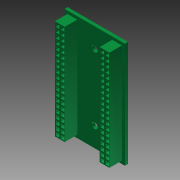
# Autodesk Inventor part: mbed breakout board
Saved by Autodesk Inventor 2012 (Build 160160000, 160)
## iProperties
Created: 2012-03-03
Part Number: mbed breakout board
Material: Default
Document SubType Name: Modeling
Designer: Lauszus
Density: 1 g/cm^3
Author: Lauszus
Autodesk Inventor part; units mm, degrees
ref_plane "YZ Plane" through (0, 0, 0) normal (1, 0, 0) x (0, 1, 0)
ref_plane "XZ Plane" through (0, 0, 0) normal (0, 1, 0) x (-1, 0, 0)
ref_plane "XY Plane" through (0, 0, 0) normal (0, 0, 1) x (1, 0, 0)
sketch "Sketch1" plane through (0, 0, 0) normal (0, 0, 1) x (1, 0, 0)
  line L0 (-19.1815, 31.3375) -> (11.6785, 31.3375)
  line L1 (11.6785, 31.3375) -> (11.6785, -22.6377)
  line L2 (11.6785, -22.6377) -> (-19.1815, -22.6377)
  line L3 (-19.1815, -22.6377) -> (-19.1815, 31.3375)
  line L4 (-17.6815, 29.8375) -> (-12.6815, 29.8375)
  line L5 (-12.6815, 29.8375) -> (-12.6815, -21.1377)
  line L6 (-12.6815, -21.1377) -> (-17.6815, -21.1377)
  line L7 (-17.6815, -21.1377) -> (-17.6815, 29.8375)
  line L8 (-17.1815, -20.6377) -> (-15.4815, -20.6377)
  line L9 (-15.4815, -20.6377) -> (-15.4815, -18.9377)
  line L10 (-15.4815, -18.9377) -> (-17.1815, -18.9377)
  line L11 (-17.1815, -18.9377) -> (-17.1815, -20.6377)
  line L12 (-14.6415, -20.6377) -> (-12.9415, -20.6377)
  line L13 (-12.9415, -20.6377) -> (-12.9415, -18.9377)
  line L14 (-12.9415, -18.9377) -> (-14.6415, -18.9377)
  line L15 (-14.6415, -18.9377) -> (-14.6415, -20.6377)
  line L16 (-17.1815, -18.0977) -> (-15.4815, -18.0977)
  line L17 (-15.4815, -18.0977) -> (-15.4815, -16.3977)
  line L18 (-15.4815, -16.3977) -> (-17.1815, -16.3977)
  line L19 (-17.1815, -16.3977) -> (-17.1815, -18.0977)
  line L20 (-14.6415, -18.0977) -> (-12.9415, -18.0977)
  line L21 (-12.9415, -18.0977) -> (-12.9415, -16.3977)
  line L22 (-12.9415, -16.3977) -> (-14.6415, -16.3977)
  line L23 (-14.6415, -16.3977) -> (-14.6415, -18.0977)
  line L24 (-17.1815, -15.5577) -> (-15.4815, -15.5577)
  line L25 (-15.4815, -15.5577) -> (-15.4815, -13.8577)
  line L26 (-15.4815, -13.8577) -> (-17.1815, -13.8577)
  line L27 (-17.1815, -13.8577) -> (-17.1815, -15.5577)
  line L28 (-14.6415, -15.5577) -> (-12.9415, -15.5577)
  line L29 (-12.9415, -15.5577) -> (-12.9415, -13.8577)
  line L30 (-12.9415, -13.8577) -> (-14.6415, -13.8577)
  line L31 (-14.6415, -13.8577) -> (-14.6415, -15.5577)
  line L32 (-12.9415, -11.3177) -> (-14.6415, -11.3177)
  line L33 (-12.9415, -13.0177) -> (-12.9415, -11.3177)
  line L34 (-14.6415, -11.3177) -> (-14.6415, -13.0177)
  line L35 (-14.6415, -13.0177) -> (-12.9415, -13.0177)
  line L36 (-17.1815, -13.0177) -> (-15.4815, -13.0177)
  line L37 (-15.4815, -13.0177) -> (-15.4815, -11.3177)
  line L38 (-15.4815, -11.3177) -> (-17.1815, -11.3177)
  line L39 (-17.1815, -11.3177) -> (-17.1815, -13.0177)
  line L40 (-17.1815, -10.4777) -> (-15.4815, -10.4777)
  line L41 (-15.4815, -10.4777) -> (-15.4815, -8.7777)
  line L42 (-15.4815, -8.7777) -> (-17.1815, -8.7777)
  line L43 (-17.1815, -8.7777) -> (-17.1815, -10.4777)
  line L44 (-14.6415, -10.4777) -> (-12.9415, -10.4777)
  line L45 (-12.9415, -10.4777) -> (-12.9415, -8.7777)
  line L46 (-12.9415, -8.7777) -> (-14.6415, -8.7777)
  line L47 (-14.6415, -8.7777) -> (-14.6415, -10.4777)
  line L48 (-12.9415, -6.2377) -> (-14.6415, -6.2377)
  line L49 (-12.9415, -7.9377) -> (-12.9415, -6.2377)
  line L50 (-14.6415, -6.2377) -> (-14.6415, -7.9377)
  line L51 (-14.6415, -7.9377) -> (-12.9415, -7.9377)
  line L52 (-17.1815, -7.9377) -> (-15.4815, -7.9377)
  line L53 (-15.4815, -7.9377) -> (-15.4815, -6.2377)
  line L54 (-15.4815, -6.2377) -> (-17.1815, -6.2377)
  line L55 (-17.1815, -6.2377) -> (-17.1815, -7.9377)
  line L56 (-17.1815, -5.3977) -> (-15.4815, -5.3977)
  line L57 (-15.4815, -5.3977) -> (-15.4815, -3.6977)
  line L58 (-15.4815, -3.6977) -> (-17.1815, -3.6977)
  line L59 (-17.1815, -3.6977) -> (-17.1815, -5.3977)
  line L60 (-14.6415, -5.3977) -> (-12.9415, -5.3977)
  line L61 (-12.9415, -5.3977) -> (-12.9415, -3.6977)
  line L62 (-12.9415, -3.6977) -> (-14.6415, -3.6977)
  line L63 (-14.6415, -3.6977) -> (-14.6415, -5.3977)
  line L64 (-12.9415, -1.1577) -> (-14.6415, -1.1577)
  line L65 (-12.9415, -2.8577) -> (-12.9415, -1.1577)
  line L66 (-14.6415, -1.1577) -> (-14.6415, -2.8577)
  line L67 (-14.6415, -2.8577) -> (-12.9415, -2.8577)
  line L68 (-17.1815, -2.8577) -> (-15.4815, -2.8577)
  line L69 (-15.4815, -2.8577) -> (-15.4815, -1.1577)
  line L70 (-15.4815, -1.1577) -> (-17.1815, -1.1577)
  line L71 (-17.1815, -1.1577) -> (-17.1815, -2.8577)
  line L72 (-17.1815, -0.3177) -> (-15.4815, -0.3177)
  line L73 (-15.4815, -0.3177) -> (-15.4815, 1.3823)
  line L74 (-15.4815, 1.3823) -> (-17.1815, 1.3823)
  line L75 (-17.1815, 1.3823) -> (-17.1815, -0.3177)
  line L76 (-14.6415, -0.3177) -> (-12.9415, -0.3177)
  line L77 (-12.9415, -0.3177) -> (-12.9415, 1.3823)
  line L78 (-12.9415, 1.3823) -> (-14.6415, 1.3823)
  line L79 (-14.6415, 1.3823) -> (-14.6415, -0.3177)
  line L80 (-12.9415, 3.9223) -> (-14.6415, 3.9223)
  line L81 (-12.9415, 2.2223) -> (-12.9415, 3.9223)
  line L82 (-14.6415, 3.9223) -> (-14.6415, 2.2223)
  line L83 (-14.6415, 2.2223) -> (-12.9415, 2.2223)
  line L84 (-17.1815, 2.2223) -> (-15.4815, 2.2223)
  line L85 (-15.4815, 2.2223) -> (-15.4815, 3.9223)
  line L86 (-15.4815, 3.9223) -> (-17.1815, 3.9223)
  line L87 (-17.1815, 3.9223) -> (-17.1815, 2.2223)
  line L88 (-17.1815, 4.7623) -> (-15.4815, 4.7623)
  line L89 (-15.4815, 4.7623) -> (-15.4815, 6.4623)
  line L90 (-15.4815, 6.4623) -> (-17.1815, 6.4623)
  line L91 (-17.1815, 6.4623) -> (-17.1815, 4.7623)
  line L92 (-14.6415, 4.7623) -> (-12.9415, 4.7623)
  line L93 (-12.9415, 4.7623) -> (-12.9415, 6.4623)
  line L94 (-12.9415, 6.4623) -> (-14.6415, 6.4623)
  line L95 (-14.6415, 6.4623) -> (-14.6415, 4.7623)
  line L96 (-12.9415, 9.0023) -> (-14.6415, 9.0023)
  line L97 (-12.9415, 7.3023) -> (-12.9415, 9.0023)
  line L98 (-14.6415, 9.0023) -> (-14.6415, 7.3023)
  line L99 (-14.6415, 7.3023) -> (-12.9415, 7.3023)
  line L100 (-17.1815, 7.3023) -> (-15.4815, 7.3023)
  line L101 (-15.4815, 7.3023) -> (-15.4815, 9.0023)
  line L102 (-15.4815, 9.0023) -> (-17.1815, 9.0023)
  line L103 (-17.1815, 9.0023) -> (-17.1815, 7.3023)
  line L104 (-17.1815, 9.8423) -> (-15.4815, 9.8423)
  line L105 (-15.4815, 9.8423) -> (-15.4815, 11.5423)
  line L106 (-15.4815, 11.5423) -> (-17.1815, 11.5423)
  line L107 (-17.1815, 11.5423) -> (-17.1815, 9.8423)
  line L108 (-14.6415, 9.8423) -> (-12.9415, 9.8423)
  line L109 (-12.9415, 9.8423) -> (-12.9415, 11.5423)
  line L110 (-12.9415, 11.5423) -> (-14.6415, 11.5423)
  line L111 (-14.6415, 11.5423) -> (-14.6415, 9.8423)
  line L112 (-12.9415, 14.0823) -> (-14.6415, 14.0823)
  line L113 (-12.9415, 12.3823) -> (-12.9415, 14.0823)
  line L114 (-14.6415, 14.0823) -> (-14.6415, 12.3823)
  line L115 (-14.6415, 12.3823) -> (-12.9415, 12.3823)
  line L116 (-17.1815, 12.3823) -> (-15.4815, 12.3823)
  line L117 (-15.4815, 12.3823) -> (-15.4815, 14.0823)
  line L118 (-15.4815, 14.0823) -> (-17.1815, 14.0823)
  line L119 (-17.1815, 14.0823) -> (-17.1815, 12.3823)
  line L120 (-17.1815, 14.9223) -> (-15.4815, 14.9223)
  line L121 (-15.4815, 14.9223) -> (-15.4815, 16.6223)
  line L122 (-15.4815, 16.6223) -> (-17.1815, 16.6223)
  line L123 (-17.1815, 16.6223) -> (-17.1815, 14.9223)
  line L124 (-14.6415, 14.9223) -> (-12.9415, 14.9223)
  line L125 (-12.9415, 14.9223) -> (-12.9415, 16.6223)
  line L126 (-12.9415, 16.6223) -> (-14.6415, 16.6223)
  line L127 (-14.6415, 16.6223) -> (-14.6415, 14.9223)
  line L128 (-12.9415, 19.1623) -> (-14.6415, 19.1623)
  line L129 (-12.9415, 17.4623) -> (-12.9415, 19.1623)
  line L130 (-14.6415, 19.1623) -> (-14.6415, 17.4623)
  line L131 (-14.6415, 17.4623) -> (-12.9415, 17.4623)
  line L132 (-17.1815, 17.4623) -> (-15.4815, 17.4623)
  line L133 (-15.4815, 17.4623) -> (-15.4815, 19.1623)
  line L134 (-15.4815, 19.1623) -> (-17.1815, 19.1623)
  line L135 (-17.1815, 19.1623) -> (-17.1815, 17.4623)
  line L136 (-17.1815, 20.0023) -> (-15.4815, 20.0023)
  line L137 (-15.4815, 20.0023) -> (-15.4815, 21.7023)
  line L138 (-15.4815, 21.7023) -> (-17.1815, 21.7023)
  line L139 (-17.1815, 21.7023) -> (-17.1815, 20.0023)
  line L140 (-14.6415, 20.0023) -> (-12.9415, 20.0023)
  line L141 (-12.9415, 20.0023) -> (-12.9415, 21.7023)
  line L142 (-12.9415, 21.7023) -> (-14.6415, 21.7023)
  line L143 (-14.6415, 21.7023) -> (-14.6415, 20.0023)
  line L144 (-12.9415, 24.2423) -> (-14.6415, 24.2423)
  line L145 (-12.9415, 22.5423) -> (-12.9415, 24.2423)
  line L146 (-14.6415, 24.2423) -> (-14.6415, 22.5423)
  line L147 (-14.6415, 22.5423) -> (-12.9415, 22.5423)
  line L148 (-17.1815, 22.5423) -> (-15.4815, 22.5423)
  line L149 (-15.4815, 22.5423) -> (-15.4815, 24.2423)
  line L150 (-15.4815, 24.2423) -> (-17.1815, 24.2423)
  line L151 (-17.1815, 24.2423) -> (-17.1815, 22.5423)
  line L152 (-17.1815, 25.0823) -> (-15.4815, 25.0823)
  line L153 (-15.4815, 25.0823) -> (-15.4815, 26.7823)
  line L154 (-15.4815, 26.7823) -> (-17.1815, 26.7823)
  line L155 (-17.1815, 26.7823) -> (-17.1815, 25.0823)
  line L156 (-14.6415, 25.0823) -> (-12.9415, 25.0823)
  line L157 (-12.9415, 25.0823) -> (-12.9415, 26.7823)
  line L158 (-12.9415, 26.7823) -> (-14.6415, 26.7823)
  line L159 (-14.6415, 26.7823) -> (-14.6415, 25.0823)
  line L160 (-12.9415, 29.3223) -> (-14.6415, 29.3223)
  line L161 (-12.9415, 27.6223) -> (-12.9415, 29.3223)
  line L162 (-14.6415, 29.3223) -> (-14.6415, 27.6223)
  line L163 (-14.6415, 27.6223) -> (-12.9415, 27.6223)
  line L164 (-17.1815, 27.6223) -> (-15.4815, 27.6223)
  line L165 (-15.4815, 27.6223) -> (-15.4815, 29.3223)
  line L166 (-15.4815, 29.3223) -> (-17.1815, 29.3223)
  line L167 (-17.1815, 29.3223) -> (-17.1815, 27.6223)
  line L168 (5.1785, 29.8375) -> (10.1785, 29.8375)
  line L169 (10.1785, 29.8375) -> (10.1785, -21.1377)
  line L170 (10.1785, -21.1377) -> (5.1785, -21.1377)
  line L171 (5.1785, -21.1377) -> (5.1785, 29.8375)
  line L172 (5.6785, -20.6377) -> (7.3785, -20.6377)
  line L173 (7.3785, -20.6377) -> (7.3785, -18.9377)
  line L174 (7.3785, -18.9377) -> (5.6785, -18.9377)
  line L175 (5.6785, -18.9377) -> (5.6785, -20.6377)
  line L176 (8.2185, -20.6377) -> (9.9185, -20.6377)
  line L177 (9.9185, -20.6377) -> (9.9185, -18.9377)
  line L178 (9.9185, -18.9377) -> (8.2185, -18.9377)
  line L179 (8.2185, -18.9377) -> (8.2185, -20.6377)
  line L180 (9.9185, -16.3977) -> (8.2185, -16.3977)
  line L181 (9.9185, -18.0977) -> (9.9185, -16.3977)
  line L182 (8.2185, -16.3977) -> (8.2185, -18.0977)
  line L183 (8.2185, -18.0977) -> (9.9185, -18.0977)
  line L184 (5.6785, -18.0977) -> (7.3785, -18.0977)
  line L185 (7.3785, -18.0977) -> (7.3785, -16.3977)
  line L186 (7.3785, -16.3977) -> (5.6785, -16.3977)
  line L187 (5.6785, -16.3977) -> (5.6785, -18.0977)
  line L188 (5.6785, -15.5577) -> (7.3785, -15.5577)
  line L189 (5.6785, -13.8577) -> (5.6785, -15.5577)
  line L190 (7.3785, -13.8577) -> (5.6785, -13.8577)
  line L191 (7.3785, -15.5577) -> (7.3785, -13.8577)
  line L192 (5.6785, -13.0177) -> (7.3785, -13.0177)
  line L193 (5.6785, -11.3177) -> (5.6785, -13.0177)
  line L194 (7.3785, -11.3177) -> (5.6785, -11.3177)
  line L195 (7.3785, -13.0177) -> (7.3785, -11.3177)
  line L196 (9.9185, -11.3177) -> (8.2185, -11.3177)
  line L197 (8.2185, -11.3177) -> (8.2185, -13.0177)
  line L198 (9.9185, -13.0177) -> (9.9185, -11.3177)
  line L199 (8.2185, -13.0177) -> (9.9185, -13.0177)
  line L200 (9.9185, -13.8577) -> (8.2185, -13.8577)
  line L201 (8.2185, -13.8577) -> (8.2185, -15.5577)
  line L202 (8.2185, -15.5577) -> (9.9185, -15.5577)
  line L203 (9.9185, -15.5577) -> (9.9185, -13.8577)
  line L204 (5.6785, -10.4777) -> (7.3785, -10.4777)
  line L205 (5.6785, -8.7777) -> (5.6785, -10.4777)
  line L206 (7.3785, -8.7777) -> (5.6785, -8.7777)
  line L207 (7.3785, -10.4777) -> (7.3785, -8.7777)
  line L208 (5.6785, -7.9377) -> (7.3785, -7.9377)
  line L209 (5.6785, -6.2377) -> (5.6785, -7.9377)
  line L210 (7.3785, -6.2377) -> (5.6785, -6.2377)
  line L211 (7.3785, -7.9377) -> (7.3785, -6.2377)
  line L212 (9.9185, -6.2377) -> (8.2185, -6.2377)
  line L213 (8.2185, -6.2377) -> (8.2185, -7.9377)
  line L214 (9.9185, -7.9377) -> (9.9185, -6.2377)
  line L215 (8.2185, -7.9377) -> (9.9185, -7.9377)
  line L216 (9.9185, -8.7777) -> (8.2185, -8.7777)
  line L217 (8.2185, -8.7777) -> (8.2185, -10.4777)
  line L218 (8.2185, -10.4777) -> (9.9185, -10.4777)
  line L219 (9.9185, -10.4777) -> (9.9185, -8.7777)
  line L220 (5.6785, -5.3977) -> (7.3785, -5.3977)
  line L221 (5.6785, -3.6977) -> (5.6785, -5.3977)
  line L222 (7.3785, -3.6977) -> (5.6785, -3.6977)
  line L223 (7.3785, -5.3977) -> (7.3785, -3.6977)
  line L224 (5.6785, -2.8577) -> (7.3785, -2.8577)
  line L225 (5.6785, -1.1577) -> (5.6785, -2.8577)
  line L226 (7.3785, -1.1577) -> (5.6785, -1.1577)
  line L227 (7.3785, -2.8577) -> (7.3785, -1.1577)
  line L228 (9.9185, -1.1577) -> (8.2185, -1.1577)
  line L229 (8.2185, -1.1577) -> (8.2185, -2.8577)
  line L230 (9.9185, -2.8577) -> (9.9185, -1.1577)
  line L231 (8.2185, -2.8577) -> (9.9185, -2.8577)
  line L232 (9.9185, -3.6977) -> (8.2185, -3.6977)
  line L233 (8.2185, -3.6977) -> (8.2185, -5.3977)
  line L234 (8.2185, -5.3977) -> (9.9185, -5.3977)
  line L235 (9.9185, -5.3977) -> (9.9185, -3.6977)
  line L236 (5.6785, -0.3177) -> (7.3785, -0.3177)
  line L237 (5.6785, 1.3823) -> (5.6785, -0.3177)
  line L238 (7.3785, 1.3823) -> (5.6785, 1.3823)
  line L239 (7.3785, -0.3177) -> (7.3785, 1.3823)
  line L240 (5.6785, 2.2223) -> (7.3785, 2.2223)
  line L241 (5.6785, 3.9223) -> (5.6785, 2.2223)
  line L242 (7.3785, 3.9223) -> (5.6785, 3.9223)
  line L243 (7.3785, 2.2223) -> (7.3785, 3.9223)
  line L244 (9.9185, 3.9223) -> (8.2185, 3.9223)
  line L245 (8.2185, 3.9223) -> (8.2185, 2.2223)
  line L246 (9.9185, 2.2223) -> (9.9185, 3.9223)
  line L247 (8.2185, 2.2223) -> (9.9185, 2.2223)
  line L248 (9.9185, 1.3823) -> (8.2185, 1.3823)
  line L249 (8.2185, 1.3823) -> (8.2185, -0.3177)
  line L250 (8.2185, -0.3177) -> (9.9185, -0.3177)
  line L251 (9.9185, -0.3177) -> (9.9185, 1.3823)
  line L252 (5.6785, 4.7623) -> (7.3785, 4.7623)
  line L253 (5.6785, 6.4623) -> (5.6785, 4.7623)
  line L254 (7.3785, 6.4623) -> (5.6785, 6.4623)
  line L255 (7.3785, 4.7623) -> (7.3785, 6.4623)
  line L256 (5.6785, 7.3023) -> (7.3785, 7.3023)
  line L257 (5.6785, 9.0023) -> (5.6785, 7.3023)
  line L258 (7.3785, 9.0023) -> (5.6785, 9.0023)
  line L259 (7.3785, 7.3023) -> (7.3785, 9.0023)
  line L260 (9.9185, 9.0023) -> (8.2185, 9.0023)
  line L261 (8.2185, 9.0023) -> (8.2185, 7.3023)
  line L262 (9.9185, 7.3023) -> (9.9185, 9.0023)
  line L263 (8.2185, 7.3023) -> (9.9185, 7.3023)
  line L264 (9.9185, 6.4623) -> (8.2185, 6.4623)
  line L265 (8.2185, 6.4623) -> (8.2185, 4.7623)
  line L266 (8.2185, 4.7623) -> (9.9185, 4.7623)
  line L267 (9.9185, 4.7623) -> (9.9185, 6.4623)
  line L268 (5.6785, 9.8423) -> (7.3785, 9.8423)
  line L269 (5.6785, 11.5423) -> (5.6785, 9.8423)
  line L270 (7.3785, 11.5423) -> (5.6785, 11.5423)
  line L271 (7.3785, 9.8423) -> (7.3785, 11.5423)
  line L272 (5.6785, 12.3823) -> (7.3785, 12.3823)
  line L273 (5.6785, 14.0823) -> (5.6785, 12.3823)
  line L274 (7.3785, 14.0823) -> (5.6785, 14.0823)
  line L275 (7.3785, 12.3823) -> (7.3785, 14.0823)
  line L276 (9.9185, 14.0823) -> (8.2185, 14.0823)
  line L277 (8.2185, 14.0823) -> (8.2185, 12.3823)
  line L278 (9.9185, 12.3823) -> (9.9185, 14.0823)
  line L279 (8.2185, 12.3823) -> (9.9185, 12.3823)
  line L280 (9.9185, 11.5423) -> (8.2185, 11.5423)
  line L281 (8.2185, 11.5423) -> (8.2185, 9.8423)
  line L282 (8.2185, 9.8423) -> (9.9185, 9.8423)
  line L283 (9.9185, 9.8423) -> (9.9185, 11.5423)
  line L284 (5.6785, 14.9223) -> (7.3785, 14.9223)
  line L285 (5.6785, 16.6223) -> (5.6785, 14.9223)
  line L286 (7.3785, 16.6223) -> (5.6785, 16.6223)
  line L287 (7.3785, 14.9223) -> (7.3785, 16.6223)
  line L288 (5.6785, 17.4623) -> (7.3785, 17.4623)
  line L289 (5.6785, 19.1623) -> (5.6785, 17.4623)
  line L290 (7.3785, 19.1623) -> (5.6785, 19.1623)
  line L291 (7.3785, 17.4623) -> (7.3785, 19.1623)
  line L292 (9.9185, 19.1623) -> (8.2185, 19.1623)
  line L293 (8.2185, 19.1623) -> (8.2185, 17.4623)
  line L294 (9.9185, 17.4623) -> (9.9185, 19.1623)
  line L295 (8.2185, 17.4623) -> (9.9185, 17.4623)
  line L296 (9.9185, 16.6223) -> (8.2185, 16.6223)
  line L297 (8.2185, 16.6223) -> (8.2185, 14.9223)
  line L298 (8.2185, 14.9223) -> (9.9185, 14.9223)
  line L299 (9.9185, 14.9223) -> (9.9185, 16.6223)
  line L300 (5.6785, 20.0023) -> (7.3785, 20.0023)
  line L301 (5.6785, 21.7023) -> (5.6785, 20.0023)
  line L302 (7.3785, 21.7023) -> (5.6785, 21.7023)
  line L303 (7.3785, 20.0023) -> (7.3785, 21.7023)
  line L304 (5.6785, 22.5423) -> (7.3785, 22.5423)
  line L305 (5.6785, 24.2423) -> (5.6785, 22.5423)
  line L306 (7.3785, 24.2423) -> (5.6785, 24.2423)
  line L307 (7.3785, 22.5423) -> (7.3785, 24.2423)
  line L308 (9.9185, 24.2423) -> (8.2185, 24.2423)
  line L309 (8.2185, 24.2423) -> (8.2185, 22.5423)
  line L310 (9.9185, 22.5423) -> (9.9185, 24.2423)
  line L311 (8.2185, 22.5423) -> (9.9185, 22.5423)
  line L312 (9.9185, 21.7023) -> (8.2185, 21.7023)
  line L313 (8.2185, 21.7023) -> (8.2185, 20.0023)
  line L314 (8.2185, 20.0023) -> (9.9185, 20.0023)
  line L315 (9.9185, 20.0023) -> (9.9185, 21.7023)
  line L316 (5.6785, 25.0823) -> (7.3785, 25.0823)
  line L317 (5.6785, 26.7823) -> (5.6785, 25.0823)
  line L318 (7.3785, 26.7823) -> (5.6785, 26.7823)
  line L319 (7.3785, 25.0823) -> (7.3785, 26.7823)
  line L320 (5.6785, 27.6223) -> (7.3785, 27.6223)
  line L321 (5.6785, 29.3223) -> (5.6785, 27.6223)
  line L322 (7.3785, 29.3223) -> (5.6785, 29.3223)
  line L323 (7.3785, 27.6223) -> (7.3785, 29.3223)
  line L324 (9.9185, 29.3223) -> (8.2185, 29.3223)
  line L325 (8.2185, 29.3223) -> (8.2185, 27.6223)
  line L326 (9.9185, 27.6223) -> (9.9185, 29.3223)
  line L327 (8.2185, 27.6223) -> (9.9185, 27.6223)
  line L328 (9.9185, 26.7823) -> (8.2185, 26.7823)
  line L329 (8.2185, 26.7823) -> (8.2185, 25.0823)
  line L330 (8.2185, 25.0823) -> (9.9185, 25.0823)
  line L331 (9.9185, 25.0823) -> (9.9185, 26.7823)
  circle A0 centre (-3.7515, 21.3375) radius 1.5
  circle A1 centre (-3.7515, -12.6377) radius 1.5
  point P0 (0, 0)
  dimension "d3" = 50.9753
  dimension "d4" = 5
  dimension "d5" = 1.5
  dimension "d6" = 1.5
  dimension "d7" = 1.7
  dimension "d8" = 1.7
  dimension "d9" = 2.54
  dimension "d10" = 1.7
  dimension "d11" = 1.7
  dimension "d12" = 0.5
  dimension "d13" = 0.5
  dimension "d14" = 0.5
  dimension "d15" = 1.7
  dimension "d16" = 1.7
  dimension "d17" = 2.54
  dimension "d18" = 1.7
  dimension "d19" = 1.7
  dimension "d21" = 2.54
  dimension "d22" = 2.54
  dimension "d23" = 0.5
  dimension "d26" = 5.08
  dimension "d33" = 22.86
  dimension "d38" = 1.5
  dimension "d39" = 1.5
  dimension "d40" = 15.43
  dimension "d41" = 15.43
  dimension "d42" = 10
  dimension "d43" = 10
  dimension "d44" = 3
  dimension "d45" = 3
  constraints: 664 end point, 12 parallel, 7 horizontal, 6 perpendicular, 2 centre point, 1 vertical, 616 other
  measures "d3" distance of L4.end L5.end
  measures "d4" distance of L4.start L4.end
  measures "d5" distance between parallel lines of L2 L6
  measures "d6" distance between parallel lines of L3 L7
  measures "d7" distance of L10.end L8.start
  measures "d8" distance of L9.end L10.end
  measures "d9" distance between parallel lines of L11 L15
  measures "d10" distance of L14.end L12.start
  measures "d11" distance of L13.end L14.end
  measures "d12" distance between parallel lines of L7 L11
  measures "d13" distance between parallel lines of L6 L8
  measures "d14" distance between parallel lines of L6 L12
  measures "d15" distance of L18.end L16.start
  measures "d16" distance of L17.end L18.end
  measures "d17" distance between parallel lines of L19 L23
  measures "d18" distance of L22.end L23.end
  measures "d19" distance of L22.start L22.end
  measures "d21" distance between parallel lines of L8 L16
  measures "d22" distance between parallel lines of L12 L20
  measures "d23" distance between parallel lines of L7 L19
  measures "d26" distance of L8.start L24.start
  measures "d33" distance of L27.start L189.start
  measures "d38" distance between parallel lines of L1 L169
  measures "d39" distance between parallel lines of L4 L0
  measures "d40" distance from line of L3 A0.centre
  measures "d41" distance from line of L3 A1.centre
  measures "d42" distance from line of L0 A0.centre
  measures "d43" distance from line of A1.centre L2
  measures "d44" diameter of A0
  measures "d45" diameter of A1
extrude "Extrusion1" add sketch "Sketch1" along normal blind 1.6 contours L0 L1 L2 L3 | L4 L5 L6 L7 | L11 L10 L9 L8 | L15 L14 L13 L12 | L19 L18 L17 L16 | L23 L22 L21 L20 | L27 L26 L25 L24 | L31 L30 L29 L28 | L33 L35 L34 L32 | L39 L38 L37 L36 | L43 L42 L41 L40 | L47 L46 L45 L44 | L49 L51 L50 L48 | L55 L54 L53 L52 | L59 L58 L57 L56 | L63 L62 L61 L60 | L65 L67 L66 L64 | L71 L70 L69 L68 | L75 L74 L73 L72 | L79 L78 L77 L76 | L81 L83 L82 L80 | L87 L86 L85 L84 | L91 L90 L89 L88 | L95 L94 L93 L92 | L97 L99 L98 L96 | L103 L102 L101 L100 | L107 L106 L105 L104 | L111 L110 L109 L108 | L113 L115 L114 L112 | L119 L118 L117 L116 | L123 L122 L121 L120 | L127 L126 L125 L124 | L129 L131 L130 L128 | L135 L134 L133 L132 | L139 L138 L137 L136 | L143 L142 L141 L140 | L145 L147 L146 L144 | L151 L150 L149 L148 | L155 L154 L153 L152 | L159 L158 L157 L156 | L161 L163 L162 L160 | L167 L166 L165 L164 | L168 L169 L170 L171 | L175 L174 L173 L172 | L179 L178 L177 L176 | L181 L183 L182 L180 | L187 L186 L185 L184 | L189 L190 L191 L188 | L193 L194 L195 L192 | L198 L199 L197 L196 | L203 L202 L201 L200 | L205 L206 L207 L204 | L209 L210 L211 L208 | L214 L215 L213 L212 | L219 L218 L217 L216 | L221 L222 L223 L220 | L225 L226 L227 L224 | L230 L231 L229 L228 | L235 L234 L233 L232 | L237 L238 L239 L236 | L241 L242 L243 L240 | L246 L247 L245 L244 | L251 L250 L249 L248 | L253 L254 L255 L252 | L257 L258 L259 L256 | L262 L263 L261 L260 | L267 L266 L265 L264 | L269 L270 L271 L268 | L273 L274 L275 L272 | L278 L279 L277 L276 | L283 L282 L281 L280 | L285 L286 L287 L284 | L289 L290 L291 L288 | L294 L295 L293 L292 | L299 L298 L297 L296 | L301 L302 L303 L300 | L305 L306 L307 L304 | L310 L311 L309 L308 | L315 L314 L313 L312 | L317 L318 L319 L316 | L321 L322 L323 L320 | L326 L327 L325 L324 | L331 L330 L329 L328
extrude "Extrusion2" add sketch "Sketch1" along normal blind 8 contours L4 L5 L6 L7 | L168 L169 L170 L171
body "Solid1"
